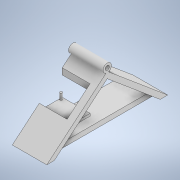
# Autodesk Inventor part: roof_foot
Saved by Autodesk Inventor 2021 (Build 250183000, 183)
## iProperties
Created: 2021-08-17
Part Number: roof_foot
Material: Generisch
Document SubType Name: Modeling
Designer: Tilman
Density: 1 g/cm^3
Appearance: Vorgabe
Author: Tilman
Autodesk Inventor part; units mm, degrees
ref_plane "YZ Plane" through (0, 0, 0) normal (1, 0, 0) x (0, 1, 0)
ref_plane "XZ Plane" through (0, 0, 0) normal (0, 1, 0) x (-1, 0, 0)
sketch "Skizze1" plane through (0, 0, 0) normal (1, 0, 0) x (0, 1, 0)
  line L0 (0, 0) -> (0, -100)
  line L1 (0, -100) -> (41.1159, -51)
  line L2 (0, 0) -> (41.1159, -49)
  circle A0 centre (44.47, -50) radius 3.5
  circle A1 centre (44.47, -50) radius 1.75
  dimension "d0" = 40
  dimension "d1" = 3.5
  dimension "d2" = 7
  dimension "d3" = 2
  dimension "d4" = 100
  constraints: 6 end point, 2 centre point, 2 point on circle, 1 coincident, 1 equal length, 1 vertical, 1 vertical alignment
  measures "d0" angle of L0 L2
  measures "d1" diameter of A1
  measures "d2" diameter of A0
  measures "d3" distance of L1.end L2.end
  measures "d4" distance of L0.start L0.end
extrude "Extrusion1" add sketch "Skizze1" along normal blind 28.5
sketch "Skizze2" plane through (0, 0, -100) normal (0, -1, 0) x (1, 0, 0)
  line L0 (0, 100) -> (0, 0) projected
  line L1 (0, 0) -> (28.5, 0) projected
  line L2 (28.5, 100) -> (28.5, 0) projected
  line L3 (0, 100) -> (28.5, 100) projected
extrude "Extrusion2" add sketch "Skizze2" along normal blind 5
sketch "Skizze3" plane through (28.5, 0, 0) normal (1, 0, 0) x (0, 0, -1)
  line L0 (100, 0) -> (51, 41.1159) projected
  arc A0 (51, 41.1159) -> (49, 41.1159) centre (50, 44.47) ccw projected
  line L1 (49, 41.1159) -> (0, 0) projected
  line L2 (0, 0) -> (0, -5) projected
  line L3 (100, -5) -> (0, -5) projected
  line L4 (100, 0) -> (100, -5) projected
  circle A1 centre (50, 44.47) radius 1.75 projected
  line L5 (49, 41.1159) -> (0, 0) projected
  line L6 (0, 0) -> (100, 0)
  line L7 (0, 0) -> (0, -5) projected
  line L8 (0, -2.5) -> (100, -2.5)
  constraints: 4 end point, 2 midpoint, 1 horizontal
extrude "Extrusion3" cut sketch "Skizze3" against normal blind 24 contours L4 L8 L2 L6
sketch "Skizze4" plane through (28.5, 0, 0) normal (1, 0, 0) x (0, 0, -1)
  line L0 (0, 0) -> (100, 0) projected
  line L1 (100, -5) -> (0, -5) projected
  line L2 (0, 0) -> (13.75, 0)
  line L3 (13.75, 0) -> (13.75, -5)
  line L4 (13.75, -5) -> (0, -5)
  line L5 (0, -5) -> (0, 0)
  line L6 (100, 0) -> (51, 41.1159) projected
  line L7 (100, 0) -> (86.25, 0)
  line L8 (86.25, 0) -> (86.25, -5)
  line L9 (86.25, -5) -> (100, -5)
  line L10 (100, -5) -> (100, 0)
  dimension "d11" = 72.5
  constraints: 16 end point, 4 parallel, 2 horizontal, 2 perpendicular, 2 point on line, 1 collinear
  measures "d11" distance between parallel lines of L8 L3
extrude "Extrusion4" cut sketch "Skizze4" against normal through all contours L0 L3 L1 L5 | L0 L10 L1 L8
sketch "Skizze5" plane through (28.5, 0, 0) normal (1, 0, 0) x (0, 0, -1)
  line L0 (86.25, -5) -> (86.25, -2.5) projected
  line L1 (86.25, -2.5) -> (13.75, -2.5) projected
  line L2 (13.75, -2.5) -> (13.75, -5) projected
  line L3 (86.25, -5) -> (13.75, -5) projected
  point P0 (0, 0)
extrude "Extrusion5" cut sketch "Skizze5" against normal blind 14.5
ref_plane "Arbeitsebene1" through (26.5, 0, 0) normal (1, 0, 0) x (0, 0, -1)
sketch "Skizze6" plane through (26.5, 0, 0) normal (1, 0, 0) x (0, 0, -1)
  line L0 (49, 41.1159) -> (0, 0) projected
  line L1 (100, 0) -> (51, 41.1159) projected
  line L2 (13.75, 0) -> (0, 0) projected
  line L3 (13.75, 0) -> (86.25, 0) projected
  line L4 (100, 0) -> (86.25, 0) projected
  line L5 (3.1114, 0) -> (50, 39.3442)
  line L6 (50, 39.3442) -> (96.8886, 0)
  circle A0 centre (50, 44.47) radius 1.75 projected
  dimension "d17" = 2
  constraints: 4 end point, 2 point on line, 1 equal length, 1 parallel, 1 vertical alignment
  measures "d17" distance between parallel lines of L0 L5
extrude "Extrusion6" cut sketch "Skizze6" against normal blind 3.5 contours L2 L5 L6 L4 L3
sketch "Skizze7" plane through (23, 0, 0) normal (1, 0, 0) x (0, 0, -1)
  line L0 (96.8886, 0) -> (3.1114, 0) projected
  line L1 (50, 39.3442) -> (96.8886, 0) projected
  line L2 (3.1114, 0) -> (50, 39.3442) projected
  line L3 (96.8886, 0) -> (3.1114, 0) projected
  line L4 (6.2229, 0) -> (50, 36.7334)
  line L5 (50, 36.7334) -> (93.7771, 0)
  line L6 (100, 0) -> (86.25, 0) projected
  point P0 (0, 0)
  dimension "d20" = 2
  constraints: 4 end point, 2 point on line, 1 equal length, 1 parallel, 1 vertical alignment
  measures "d20" distance between parallel lines of L2 L4
extrude "Extrusion7" cut sketch "Skizze7" along normal through all contours L0 L4 L5
sketch "Skizze8" plane through (0, 0, 0) normal (-1, 0, 0) x (0, 0, 1)
  line L0 (-100, 0) -> (-86.25, 0) projected
  line L1 (-13.75, 0) -> (0, 0) projected
  line L2 (-13.75, 0) -> (-86.25, 0) projected
  line L3 (-49, 41.1159) -> (0, 0) projected
  line L4 (-100, 0) -> (-51, 41.1159) projected
  circle A0 centre (-50, 44.47) radius 1.75 projected
  line L5 (-93.7771, 0) -> (-96.8886, 0) projected
  line L6 (-50, 39.3442) -> (-96.8886, 0) projected
  line L7 (-92.1215, 4) -> (-7.8785, 4)
  line L8 (-3.1114, 0) -> (-50, 39.3442) projected
  line L9 (-93.7771, 0) -> (-50, 36.7334) projected
  line L10 (-50, 36.7334) -> (-6.2229, 0) projected
  point P0 (-10.9899, 4)
  point P1 (-89.0101, 4)
  dimension "d23" = 4
  constraints: 2 end point, 2 point on line, 1 horizontal
  measures "d23" distance between parallel lines of L2 L7
extrude "Extrusion8" cut sketch "Skizze8" against normal up to surface (23 mm away) contours L9 L10 L7
sketch "Skizze9" plane through (0, 0, 0) normal (-1, 0, 0) x (0, 0, 1)
  line L0 (-89.0101, 4) -> (-50, 36.7334) projected
  line L1 (-50, 36.7334) -> (-10.9899, 4) projected
  line L2 (-10.9899, 4) -> (-89.0101, 4) projected
  line L3 (-86.25, 0) -> (-86.25, -5) projected
  line L4 (-13.75, -5) -> (-86.25, -5) projected
  line L5 (-13.75, -5) -> (-13.75, 0) projected
  line L6 (-13.75, 0) -> (0, 0) projected
  line L7 (-49, 41.1159) -> (0, 0) projected
  arc A0 (-49, 41.1159) -> (-51, 41.1159) centre (-50, 44.47) ccw projected
  line L8 (-100, 0) -> (-51, 41.1159) projected
  line L9 (-100, 0) -> (-86.25, 0) projected
  circle A1 centre (-50, 44.47) radius 1.75 projected
  line L10 (-19.9281, 11.5) -> (-41.3116, 11.5)
  line L11 (-41.3116, 11.5) -> (-41.3116, 13.5)
  line L12 (-41.3116, 13.5) -> (-22.3116, 13.5)
  line L13 (-50, 36.7334) -> (-10.9899, 4) projected
  point P0 (-30.495, 20.3667)
  dimension "d26" = 2
  dimension "d27" = 19
  dimension "d38" = 7.5
  constraints: 6 end point, 2 perpendicular, 2 point on line, 1 horizontal
  measures "d26" distance of L10.end L11.end
  measures "d27" distance of L12.end L11.end
  measures "d38" distance between parallel lines of L2 L10
extrude "Extrusion9" add sketch "Skizze9" against normal up to surface (23 mm away) contours L1 L10 L11 L12
sketch "Skizze10" plane through (0, 13.5, -22.3116) normal (0, 1, 0) x (1, 0, 0)
  line L0 (23, 19) -> (23, 0) projected
  line L1 (0, 19) -> (23, 19) projected
  line L2 (0, 0) -> (0, 19) projected
  line L3 (23, 0) -> (0, 0) projected
  circle A0 centre (16, 17) radius 1
  circle A1 centre (1, 17) radius 1
  point P0 (0, -22.3116)
  dimension "d30" = 2
  dimension "d31" = 15
  dimension "d32" = 2
  dimension "d39" = 1
  constraints: 2 centre point, 1 equal radius, 1 horizontal alignment
  measures "d30" diameter of A0
  measures "d31" distance of A1.centre A0.centre
  measures "d32" distance from line of L1 A0.centre
  measures "d39" distance from line of L2 A1.centre
extrude "Extrusion10" cut sketch "Skizze10" along normal through all contours A1 | L0 L3 L2 L1 | A0
extrude "Extrusion11" add sketch "Skizze10" along normal blind 5 contours A1 | A0
equation "\"d32\" = d30"
